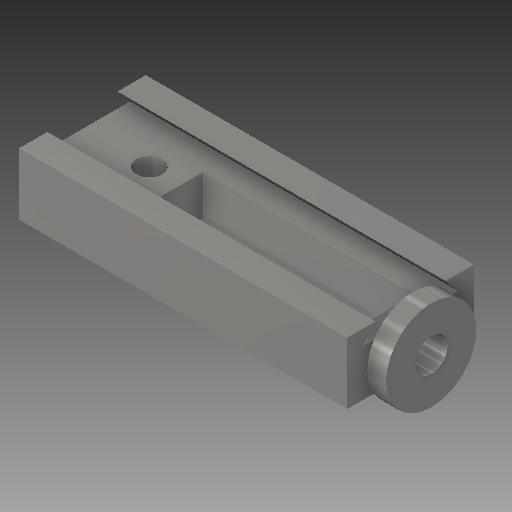
# Autodesk Inventor part: Bottom Tool Bit
Saved by Autodesk Inventor 2018 (Build 220112000, 112)
## iProperties
Created: 2017-05-07
Part Number: Bottom Tool Bit
Material: Steel, Cast
Document SubType Name: Modeling
Designer: Alex
Density: 7.85 g/cm^3
Appearance: Semi-Polished
Mass: 4401.23 g
Surface Area: 885.4 cm^2
Volume: 560.666 cm^3
Author: Alex
Autodesk Inventor part; units mm, degrees
ref_plane "YZ Plane" through (0, 0, 0) normal (1, 0, 0) x (0, 1, 0)
ref_plane "XZ Plane" through (0, 0, 0) normal (0, 1, 0) x (-1, 0, 0)
ref_plane "XY Plane" through (0, 0, 0) normal (0, 0, 1) x (1, 0, 0)
sketch "Sketch1" plane through (0, 0, 0) normal (1, 0, 0) x (0, 1, 0)
  line L0 (0, 0) -> (0, -85)
  line L1 (0, -85) -> (41.4, -85)
  line L2 (41.4, -85) -> (41.4, 0)
  line L3 (41.4, 0) -> (0, 0)
  dimension "d0" = 85
  dimension "d1" = 41.4
  constraints: 8 end point, 3 perpendicular, 1 vertical
  measures "d0" distance of L0.start L0.end
  measures "d1" distance of L0.end L1.end
extrude "Extrusion1" add sketch "Sketch1" against normal blind 220
sketch "Sketch2" plane through (0, 0, 0) normal (1, 0, 0) x (0, 0, -1)
  line L0 (0, 41.4) -> (19, 41.4)
  line L1 (10.609, 31.4) -> (19, 41.4)
  line L2 (10.609, 31.4) -> (74.391, 31.4)
  line L3 (85, 41.4) -> (66, 41.4)
  line L4 (66, 41.4) -> (74.391, 31.4)
  line L5 (19, 41.4) -> (66, 41.4)
  line L6 (0, 41.4) -> (85, 41.4) projected
  line L7 (42.5, 41.4) -> (42.5, 31.4) construction
  dimension "d4" = 19
  dimension "d8" = 19
  dimension "d61" = 50
  dimension "d63" = 50
  dimension "d64" = 10
  constraints: 14 end point, 2 midpoint, 1 collinear, 1 horizontal, 1 vertical
  measures "d4" distance of L0.start L0.end
  measures "d8" distance of L3.start L3.end
  measures "d61" angle of L0 L1
  measures "d63" angle of L3 L4
  measures "d64" distance of L7.start L7.end
extrude "Extrusion2" cut sketch "Sketch2" against normal blind 301.25
sketch "Sketch3" plane through (0, 31.4, -10.609) normal (0, 1, 0) x (1, 0, 0)
  line L0 (0, -10.609) -> (0, 74.391) projected
  line L1 (-12.6, 32) -> (-12.6, 47.1)
  line L2 (-12.6, 32) -> (-12.6, 16.9)
  line L3 (-12.6, 16.9) -> (-154.5, 16.9)
  line L4 (-154.5, 16.9) -> (-154.5, 47.1)
  line L5 (-154.5, 47.1) -> (-12.6, 47.1)
  dimension "d12" = 15.1
  dimension "d13" = 15.1
  dimension "d14" = 141.9
  constraints: 10 end point, 2 perpendicular, 1 parallel, 1 vertical
  measures "d12" distance of L1.start L1.end
  measures "d13" distance of L1.start L2.end
  measures "d14" distance of L2.end L3.end
extrude "Extrusion3" cut sketch "Sketch3" against normal blind 26.9
sketch "Sketch5" plane through (0, 0, 0) normal (1, 0, 0) x (0, 0, -1)
  line L0 (0, 41.4) -> (0, 0) projected
  line L1 (0, 0) -> (28.6, 0)
  line L2 (85, 0) -> (0, 0) projected
  line L3 (28.6, 0) -> (58.8, 0)
  line L4 (85, 41.4) -> (85, 0) projected
  line L5 (58.8, 0) -> (85, 0)
  line L6 (28.6, 0) -> (43.7, 0)
  line L7 (43.7, 0) -> (43.7, 31.4)
  line L8 (27.509, 31.4) -> (57.709, 31.4) projected
  line L9 (43.7, 31.4) -> (43.7, 26.8)
  line L10 (43.7, 26.8) -> (43.7, 14.6)
  line L11 (43.7, 26.8) -> (43.7, 15.8)
  circle A0 centre (43.7, 15.8) radius 11
  dimension "d17" = 28.6
  dimension "d18" = 30.2
  dimension "d19" = 4.6
  dimension "d21" = 11
  constraints: 16 end point, 6 point on line, 1 coincident, 1 collinear, 1 midpoint, 1 perpendicular, 1 vertical alignment, 2 other
  measures "d17" distance of L0.end L1.end
  measures "d18" distance of L1.end L3.end
  measures "d19" distance of L7.end L9.end
  measures "d21" distance of L9.end L11.end
extrude "Extrusion4" cut sketch "Sketch5" against normal blind 91.9
sketch "Sketch7" plane through (0, 0, 0) normal (1, 0, 0) x (0, 0, -1)
  circle A0 centre (43.7, 15.8) radius 11 projected
  circle A1 centre (43.7, 15.8) radius 30.2
  point P0 (0, 0)
  dimension "d24" = 60.4
  constraints: 1 centre point, 1 coincident
  measures "d24" diameter of A1
extrude "Extrusion5" add sketch "Sketch7" along normal blind 12.7
sketch "Sketch8" plane through (0, 0, -85) normal (0, 0, -1) x (-1, 0, 0)
  line L0 (220, 31.4) -> (220, 41.4) projected
  line L1 (220, 41.4) -> (220, 30.8)
  line L2 (220, 41.4) -> (220, 0) projected
  line L3 (220, 30.8) -> (136.4, 30.8)
  line L4 (154.5, 31.4) -> (12.6, 31.4) projected
  line L5 (136.4, 30.8) -> (136.4, 25.9)
  line L6 (0, 0) -> (220, 0) projected
  circle A0 centre (136.4, 25.9) radius 4.9
  dimension "d27" = 10.6
  dimension "d28" = 83.6
  dimension "d29" = 90
  dimension "d30" = 4.9
  constraints: 6 end point, 1 coincident, 1 parallel, 1 perpendicular, 1 point on line, 1 vertical alignment, 2 other
  measures "d27" distance of L0.end L1.end
  measures "d28" distance of L1.end L3.end
  measures "d29" angle of L1 L3
  measures "d30" distance of L3.end L5.end
extrude "Extrusion6" cut sketch "Sketch8" against normal blind 6
sketch "Sketch9" plane through (-220, 0, 0) normal (0, -1, 0) x (1, 0, 0)
  line L0 (0, -85) -> (0, 0) projected
  line L1 (0, -85) -> (0, -63)
  line L2 (0, -63) -> (22.3, -63)
  line L3 (0, 0) -> (0, -22.7)
  line L4 (0, -22.7) -> (22.3, -22.7)
  line L5 (22.3, -22.7) -> (22.3, -63)
  line L6 (22.3, -42.85) -> (44.45, -42.85)
  line L7 (65.5, -27.509) -> (65.5, -57.709) projected
  line L8 (22.3, -42.85) -> (44.45, -42.85) construction
  circle A0 centre (44.45, -42.85) radius 22.15
  point P0 (220, 0)
  dimension "d33" = 22
  dimension "d34" = 22.3
  dimension "d35" = 22.7
  dimension "d36" = 22.15
  dimension "d37" = 0
  constraints: 14 end point, 4 perpendicular, 2 point on line, 1 coincident, 1 collinear, 1 horizontal, 1 horizontal alignment, 1 midpoint, 2 other
  measures "d33" distance of L0.start L1.end
  measures "d34" distance of L1.end L2.end
  measures "d35" distance of L0.end L3.end
  measures "d36" distance of L6.start L6.end
  measures "d37" distance between parallel lines of L6 L8
extrude "Extrusion7" add sketch "Sketch9" along normal blind 4.6 contours A0 L7 | A0 L7
sketch "Sketch10" plane through (-175.55, -4.6, -42.85) normal (0, -1, 0) x (1, 0, 0)
  circle A0 centre (0, 0) radius 8.75
  point P0 (175.55, 42.85)
  dimension "d40" = 17.5
  constraints: 1 centre point
  measures "d40" diameter of A0
extrude "Extrusion8" cut sketch "Sketch10" against normal blind 310.85
sketch "Sketch11" plane through (-175.55, -4.6, -42.85) normal (0, -1, 0) x (1, 0, 0)
  circle A0 centre (0, 0) radius 8.75 projected
  line L0 (-8.75, 0) -> (-13.15, 0)
  line L1 (-13.15, 0) -> (-18.15, 0)
  circle A1 centre (-15.65, 0) radius 2.5
  line L2 (8.75, 0) -> (13.15, 0)
  line L3 (13.15, 0) -> (15.65, 0)
  circle A2 centre (15.65, 0) radius 2.5
  point P0 (175.55, 42.85)
  dimension "d43" = 4.4
  dimension "d44" = 5
  dimension "d45" = 4.4
  dimension "d46" = 2.5
  constraints: 8 end point, 3 horizontal, 2 horizontal alignment, 2 point on circle, 1 coincident, 1 midpoint, 1 point on line, 4 other
  measures "d43" distance of L0.start L0.end
  measures "d44" distance of L0.end L1.end
  measures "d45" distance of L2.start L2.end
  measures "d46" distance of L2.end L3.end
extrude "Extrusion9" cut sketch "Sketch11" against normal blind 3.5 contours A1 L1 | L1 A1 | A2
sketch "Sketch12" plane through (-220, 0, 0) normal (0, -1, 0) x (1, 0, 0)
  line L0 (0, 0) -> (40.7, 0)
  line L1 (220, 0) -> (0, 0) projected
  line L2 (40.7, 0) -> (40.7, -9.4)
  line L3 (40.7, -9.4) -> (40.7, -13.4)
  circle A0 centre (40.7, -13.4) radius 4
  line L4 (220, -85) -> (0, -85) projected
  line L5 (0, -85) -> (40.7, -85)
  line L6 (40.7, -85) -> (40.7, -75.6)
  line L7 (40.7, -75.6) -> (40.7, -71.6)
  circle A1 centre (40.7, -71.6) radius 4
  line L8 (0, 0) -> (70.6, 0)
  line L9 (70.6, 0) -> (70.6, -39.5)
  line L10 (70.6, -39.5) -> (70.6, -44)
  line L11 (70.6, -39.5) -> (75.1, -39.5)
  line L12 (75.1, -39.5) -> (75.1, -44)
  circle A2 centre (75.1, -44) radius 4.5
  dimension "d49" = 40.7
  dimension "d50" = 9.4
  dimension "d51" = 4
  dimension "d52" = 40.7
  dimension "d53" = 9.4
  dimension "d54" = 4
  dimension "d55" = 70.6
  dimension "d56" = 39.5
  dimension "d57" = 4.5
  dimension "d58" = 4.5
  constraints: 22 end point, 5 point on line, 4 perpendicular, 3 coincident, 2 vertical alignment, 1 horizontal, 1 horizontal alignment, 1 vertical, 6 other
  measures "d49" distance of L0.start L0.end
  measures "d50" distance of L0.end L2.end
  measures "d51" distance of L2.end L3.end
  measures "d52" distance of L4.end L5.end
  measures "d53" distance of L5.end L6.end
  measures "d54" distance of L6.end L7.end
  measures "d55" distance of L0.start L8.end
  measures "d56" distance of L8.end L9.end
  measures "d57" distance of L9.end L10.end
  measures "d58" distance of L9.end L11.end
extrude "Extrusion10" cut sketch "Sketch12" against normal blind 7 contours A0 | A2 | A1
body "Solid1"
